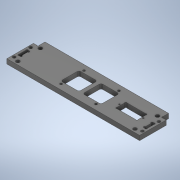
# Autodesk Inventor part: Cockpit_top_frame
Saved by Autodesk Inventor 2020.4 (Build 244396000, 396)
## iProperties
Created: 2022-01-20
Part Number: Cockpit_top_frame
Material: アセタール樹脂、黒
Document SubType Name: Modeling
Designer: Masato Kubotera
Density: 1.425 g/cm^3
Appearance: 滑らか - 黒
Author: Masato Kubotera
Autodesk Inventor part; units mm, degrees
ref_plane "YZ Plane" through (0, 0, 0) normal (1, 0, 0) x (0, 1, 0)
ref_plane "XZ Plane" through (0, 0, 0) normal (0, 1, 0) x (-1, 0, 0)
derived "Cockpit_side_frame.ipt"
sketch "スケッチ1" plane through (0, 0, 0) normal (0, 1, 0) x (-1, 0, 0)
  line L0 (-60, 36.75) -> (60, 36.75) construction
  line L1 (60, 36.75) -> (60, -36.75) construction
  line L2 (60, -36.75) -> (-60, -36.75) construction
  line L3 (-60, -36.75) -> (-60, 36.75) construction
  line L4 (-60, 36.75) -> (60, -36.75) construction
  line L5 (60, 36.75) -> (-60, -36.75) construction
  line L6 (-52.5, 6.75) -> (52.5, 6.75) construction
  line L7 (52.5, 6.75) -> (52.5, 1.75) construction
  line L8 (52.5, 1.75) -> (-52.5, 1.75) construction
  line L9 (-52.5, 1.75) -> (-52.5, 6.75) construction
  line L10 (-52.5, 6.75) -> (52.5, 1.75) construction
  line L11 (52.5, 6.75) -> (-52.5, 1.75) construction
  line L12 (0, 36.75) -> (0, -36.75) construction
  line L13 (-57.5, 34.25) -> (-52.5, 34.25) construction
  line L14 (-52.5, 34.25) -> (-52.5, -34.25) construction
  line L15 (-52.5, -34.25) -> (-57.5, -34.25) construction
  line L16 (-57.5, -34.25) -> (-57.5, 34.25) construction
  line L17 (-57.5, 34.25) -> (-52.5, -34.25) construction
  line L18 (-52.5, 34.25) -> (-57.5, -34.25) construction
  line L19 (-55, 36.75) -> (-60, 31.75)
  line L20 (-60, 0) -> (60, 0) construction
  line L21 (-46.5, 41.75) -> (32.5, 41.75) construction
  line L22 (32.5, 41.75) -> (32.5, 11.75) construction
  line L23 (32.5, 11.75) -> (-46.5, 11.75) construction
  line L24 (-46.5, 11.75) -> (-46.5, 41.75) construction
  line L25 (-46.5, 41.75) -> (32.5, 11.75) construction
  line L26 (32.5, 41.75) -> (-46.5, 11.75) construction
  line L27 (-55, -36.75) -> (-60, -31.75)
  line L28 (-60, 31.75) -> (-60, -31.75)
  line L29 (55, -36.75) -> (60, -31.75)
  line L30 (-52.5, -29.25) -> (52.5, -29.25) construction
  line L31 (52.5, -29.25) -> (52.5, -34.25) construction
  line L32 (52.5, -34.25) -> (-52.5, -34.25) construction
  line L33 (-52.5, -34.25) -> (-52.5, -29.25) construction
  line L34 (-52.5, -29.25) -> (52.5, -34.25) construction
  line L35 (52.5, -29.25) -> (-52.5, -34.25) construction
  line L36 (-25, -29.25) -> (-25, -34.25) construction
  line L37 (-55, -34.25) -> (-55, 34.25) construction
  line L38 (-57.5, 12.5) -> (-52.5, 12.5) construction
  line L39 (-57.55, 12.55) -> (-52.45, 12.55)
  line L40 (-52.45, 12.55) -> (-52.45, -12.55)
  line L41 (-52.45, -12.55) -> (-57.55, -12.55)
  line L42 (-57.55, -12.55) -> (-57.55, 12.55)
  line L43 (-57.55, 12.55) -> (-52.45, -12.55) construction
  line L44 (-52.45, 12.55) -> (-57.55, -12.55) construction
  arc A0 (-52.45, 11.0651) -> (-53.9349, 12.55) centre (-53.1925, 11.8075) ccw
  circle A1 centre (-55, 20) radius 1.6
  circle A2 centre (-55, -20) radius 1.6
  arc A3 (-53.9349, -12.55) -> (-52.45, -11.0651) centre (-53.1925, -11.8075) ccw
  line L45 (-57.5, -12.5) -> (-52.5, -12.5) construction
  arc A4 (-56.0651, 12.55) -> (-57.55, 11.0651) centre (-56.8075, 11.8075) ccw
  arc A5 (-57.55, -11.0651) -> (-56.0651, -12.55) centre (-56.8075, -11.8075) ccw
  line L46 (-52.5, -31.75) -> (52.5, -31.75) construction
  line L47 (-25.05, -34.3) -> (-25.05, -29.2)
  line L48 (-25.05, -29.2) -> (25.05, -29.2)
  circle A6 centre (-32.5, -31.75) radius 1.6
  circle A7 centre (32.5, -31.75) radius 1.6
  line L49 (25, -29.25) -> (25, -34.25) construction
  line L50 (52.5, 36.75) -> (57.5, 36.75) construction
  line L51 (57.5, 36.75) -> (57.5, -34.25) construction
  line L52 (57.5, -34.25) -> (52.5, -34.25) construction
  line L53 (52.5, -34.25) -> (52.5, 36.75) construction
  line L54 (52.5, 36.75) -> (57.5, -34.25) construction
  line L55 (57.5, 36.75) -> (52.5, -34.25) construction
  line L56 (52.5, 1.25) -> (57.5, 1.25) construction
  line L57 (52.5, -11.25) -> (57.5, -11.25) construction
  line L58 (55, -34.25) -> (55, 36.75) construction
  circle A8 centre (55, -18.75) radius 1.6
  line L59 (60, -11.3) -> (52.45, -11.3)
  line L60 (52.45, -11.3) -> (52.45, 13.8)
  arc A9 (52.45, -9.8151) -> (53.9349, -11.3) centre (53.1925, -10.5575) ccw
  line L61 (60, 13.8) -> (52.45, 13.8)
  arc A10 (53.9349, 13.8) -> (52.45, 12.3151) centre (53.1925, 13.0575) ccw
  line L62 (52.5, 13.75) -> (57.5, 13.75) construction
  circle A11 centre (55, 21.25) radius 1.6
  arc A12 (-23.5651, -29.2) -> (-25.05, -30.6849) centre (-24.3075, -29.9425) ccw
  arc A13 (25.05, -30.6849) -> (23.5651, -29.2) centre (24.3075, -29.9425) ccw
  circle A14 centre (-55, 20) radius 3
  circle A15 centre (-32.5, -31.75) radius 3
  circle A16 centre (-55, -20) radius 3
  circle A17 centre (32.5, -31.75) radius 3
  line L63 (25.05, -34.3) -> (25.05, -29.2)
  line L64 (25.05, 6.8) -> (-25.05, 6.8)
  line L65 (-25.05, 6.8) -> (-25.05, 1.7)
  line L66 (-25.05, 1.7) -> (25.05, 1.7)
  line L67 (25.05, 1.7) -> (25.05, 6.8)
  line L68 (25.05, 6.8) -> (-25.05, 1.7) construction
  line L69 (-25.05, 6.8) -> (25.05, 1.7) construction
  line L70 (-25, 6.75) -> (-25, 1.75) construction
  arc A18 (-23.5651, 6.8) -> (-25.05, 5.3151) centre (-24.3075, 6.0575) ccw
  line L71 (52.5, 4.25) -> (-52.5, 4.25) construction
  circle A19 centre (-32.5, 4.25) radius 1.6
  line L72 (25, 6.75) -> (25, 1.75) construction
  arc A20 (25.05, 5.3151) -> (23.5651, 6.8) centre (24.3075, 6.0575) ccw
  circle A21 centre (32.5, 4.25) radius 1.6
  arc A22 (-25.05, 3.1849) -> (-23.5651, 1.7) centre (-24.3075, 2.4425) ccw
  arc A23 (23.5651, 1.7) -> (25.05, 3.1849) centre (24.3075, 2.4425) ccw
  line L73 (60, 31.75) -> (60, 13.8)
  line L74 (60, -11.3) -> (60, -31.75)
  circle A24 centre (-32.5, 4.25) radius 3
  circle A25 centre (55, -18.75) radius 3
  circle A26 centre (55, 21.25) radius 3
  circle A27 centre (32.5, 4.25) radius 3
  line L75 (60, 31.75) -> (60, 39.25)
  line L76 (21, 36.75) -> (-55, 36.75)
  line L77 (60, 39.25) -> (57.5, 41.75)
  line L78 (57.5, 41.75) -> (50, 41.75)
  line L79 (50, 41.75) -> (50, 36.75)
  line L80 (50, 36.75) -> (40.5, 36.75)
  line L81 (40.5, 36.75) -> (40.5, 41.75)
  line L82 (40.5, 41.75) -> (30.5, 41.75)
  line L83 (30.5, 41.75) -> (30.5, 36.75)
  line L84 (30.5, 36.75) -> (21, 36.75)
  line L85 (21, 36.75) -> (21, 36.75)
  circle A28 centre (-45, 4.25) radius 1.75
  line L86 (35.5, 41.75) -> (35.5, 36.75) construction
  line L87 (37.9, -8.6) -> (47.1, -8.6) construction
  line L88 (47.1, -8.6) -> (47.1, -22.4) construction
  line L89 (47.1, -22.4) -> (37.9, -22.4) construction
  line L90 (37.9, -22.4) -> (37.9, -8.6) construction
  line L91 (37.9, -8.6) -> (47.1, -22.4) construction
  line L92 (47.1, -8.6) -> (37.9, -22.4) construction
  line L93 (37.2, -7.95) -> (47.8, -7.95) construction
  line L94 (47.8, -7.95) -> (47.8, -23.05) construction
  line L95 (47.8, -23.05) -> (37.2, -23.05) construction
  line L96 (37.2, -23.05) -> (37.2, -7.95) construction
  line L97 (37.2, -7.95) -> (47.8, -23.05) construction
  line L98 (47.8, -7.95) -> (37.2, -23.05) construction
  line L99 (42.5, -7.95) -> (42.5, -23.05) construction
  line L100 (47.8, -15.5) -> (37.2, -15.5) construction
  line L101 (38.6349, -7.9) -> (46.3651, -7.9)
  line L102 (37.15, -9.3849) -> (37.15, -21.6151)
  line L103 (39.3349, -8.55) -> (45.6651, -8.55)
  line L104 (37.85, -10.0349) -> (37.85, -20.9651)
  arc A29 (38.6349, -7.9) -> (37.15, -9.3849) centre (37.8925, -8.6425) ccw
  arc A30 (39.3349, -8.55) -> (37.85, -10.0349) centre (38.5925, -9.2925) ccw
  arc A31 (47.85, -9.3849) -> (46.3651, -7.9) centre (47.1075, -8.6425) ccw
  arc A32 (47.15, -10.0349) -> (45.6651, -8.55) centre (46.4075, -9.2925) ccw
  line L105 (38.6349, -23.1) -> (46.3651, -23.1)
  line L106 (39.3349, -22.45) -> (45.6651, -22.45)
  arc A33 (37.85, -20.9651) -> (39.3349, -22.45) centre (38.5925, -21.7075) ccw
  arc A34 (37.15, -21.6151) -> (38.6349, -23.1) centre (37.8925, -22.3575) ccw
  arc A35 (46.3651, -23.1) -> (47.85, -21.6151) centre (47.1075, -22.3575) ccw
  arc A36 (45.6651, -22.45) -> (47.15, -20.9651) centre (46.4075, -21.7075) ccw
  line L107 (47.15, -10.0349) -> (47.15, -20.9651)
  line L108 (47.85, -9.3849) -> (47.85, -21.6151)
  line L109 (-45.5, -4.25) -> (10.5, -4.25)
  line L110 (12.5, -6.25) -> (12.5, -22.25)
  line L111 (10.5, -24.25) -> (-45.5, -24.25)
  line L112 (-47.5, -22.25) -> (-47.5, -6.25)
  line L113 (-47.5, -4.25) -> (12.5, -24.25) construction
  line L114 (12.5, -4.25) -> (-47.5, -24.25) construction
  arc A37 (-45.5, -4.25) -> (-47.5, -6.25) centre (-45.5, -6.25) ccw
  arc A38 (-47.5, -22.25) -> (-45.5, -24.25) centre (-45.5, -22.25) ccw
  arc A39 (10.5, -24.25) -> (12.5, -22.25) centre (10.5, -22.25) ccw
  arc A40 (12.5, -6.25) -> (10.5, -4.25) centre (10.5, -6.25) ccw
  line L115 (26.5, 36.75) -> (26.5, 32.75) construction
  line L116 (24.5, 32.75) -> (28.5, 32.75) construction
  line L117 (28.5, 32.75) -> (28.5, 36.75) construction
  line L118 (24.5, 32.75) -> (24.5, 36.75) construction
  line L119 (42.5, 32.75) -> (42.5, 36.75) construction
  line L120 (44.5, 36.75) -> (44.5, 32.75) construction
  line L121 (46.5, 32.75) -> (42.5, 32.75) construction
  line L122 (46.5, 32.75) -> (46.5, 36.75) construction
  arc A41 (48.5151, 36.75) -> (50, 38.2349) centre (49.2575, 37.4925) ccw
  arc A42 (29.0151, 36.75) -> (30.5, 38.2349) centre (29.7575, 37.4925) ccw
  arc A43 (40.5, 38.2349) -> (41.9849, 36.75) centre (41.2425, 37.4925) ccw
  line L123 (30.5, 36.75) -> (40.5, 36.75)
  line L124 (60, -36.75) -> (60, -79.25)
  line L125 (60, -79.25) -> (14, -79.25)
  line L126 (9, -74.25) -> (9, -36.75)
  arc A44 (-25.05, -32.8151) -> (-23.5651, -34.3) centre (-24.3075, -33.5575) ccw
  arc A45 (23.5651, -34.3) -> (25.05, -32.8151) centre (24.3075, -33.5575) ccw
  line L127 (60, -36.75) -> (60, -31.75)
  line L128 (-25.05, -34.3) -> (25.05, -34.3)
  line L129 (-55, -36.75) -> (9, -36.75)
  line L130 (16.5, -48.75) -> (50.5, -48.75) construction
  line L131 (50.5, -48.75) -> (50.5, -71.75) construction
  line L132 (50.5, -71.75) -> (16.5, -71.75) construction
  line L133 (16.5, -71.75) -> (16.5, -48.75) construction
  line L134 (16.5, -48.75) -> (50.5, -71.75) construction
  line L135 (50.5, -48.75) -> (16.5, -71.75) construction
  line L136 (14, -45.5) -> (16.5, -45.5) construction
  line L137 (16.5, -45.5) -> (16.5, -60.5) construction
  line L138 (16.5, -60.5) -> (14, -60.5) construction
  line L139 (14, -60.5) -> (14, -45.5) construction
  line L140 (14, -45.5) -> (16.5, -60.5) construction
  line L141 (16.5, -45.5) -> (14, -60.5) construction
  line L142 (13.95, -45.45) -> (16.55, -45.45)
  line L143 (16.55, -45.45) -> (16.55, -60.55)
  line L144 (16.55, -60.55) -> (13.95, -60.55)
  line L145 (13.95, -60.55) -> (13.95, -45.45)
  line L146 (13.95, -45.45) -> (16.55, -60.55) construction
  line L147 (16.55, -45.45) -> (13.95, -60.55) construction
  line L148 (15.25, -45.5) -> (15.25, -60.5) construction
  line L149 (14, -53) -> (16.5, -53) construction
  arc A46 (15.4349, -45.45) -> (13.95, -46.9349) centre (14.6925, -46.1925) ccw
  arc A47 (16.55, -47.55) -> (16.55, -45.45) centre (16.55, -46.5) ccw
  arc A48 (13.95, -59.0651) -> (15.4349, -60.55) centre (14.6925, -59.8075) ccw
  arc A49 (16.55, -60.55) -> (16.55, -58.45) centre (16.55, -59.5) ccw
  line L150 (11.5, -34.25) -> (16.5, -34.25) construction
  line L151 (16.5, -34.25) -> (16.5, -71.75) construction
  line L152 (16.5, -71.75) -> (11.5, -71.75) construction
  line L153 (11.5, -71.75) -> (11.5, -34.25) construction
  line L154 (11.5, -34.25) -> (16.5, -71.75) construction
  line L155 (16.5, -34.25) -> (11.5, -71.75) construction
  circle A50 centre (14, -39.5) radius 1.6
  line L156 (14, -34.25) -> (14, -71.75) construction
  circle A51 centre (14, -66.5) radius 1.6
  line L157 (14, -79.25) -> (9, -74.25)
  circle A52 centre (14, -39.5) radius 3
  circle A53 centre (14, -66.5) radius 3
  line L158 (11.5, -71.75) -> (50, -71.75) construction
  line L159 (50, -71.75) -> (50, -76.75) construction
  line L160 (50, -76.75) -> (11.5, -76.75) construction
  line L161 (11.5, -76.75) -> (11.5, -71.75) construction
  line L162 (11.5, -71.75) -> (50, -76.75) construction
  line L163 (50, -71.75) -> (11.5, -76.75) construction
  line L164 (30.75, -76.75) -> (30.75, -71.75) construction
  line L165 (11.5, -74.25) -> (50, -74.25) construction
  line L166 (25.75, -71.75) -> (35.75, -71.75) construction
  line L167 (35.75, -71.75) -> (35.75, -74.25) construction
  line L168 (35.75, -74.25) -> (25.75, -74.25) construction
  line L169 (25.75, -74.25) -> (25.75, -71.75) construction
  line L170 (25.75, -71.75) -> (35.75, -74.25) construction
  line L171 (35.75, -71.75) -> (25.75, -74.25) construction
  line L172 (25.7, -71.7) -> (35.8, -71.7)
  line L173 (35.8, -71.7) -> (35.8, -74.3)
  line L174 (35.8, -74.3) -> (25.7, -74.3)
  line L175 (25.7, -74.3) -> (25.7, -71.7)
  line L176 (25.7, -71.7) -> (35.8, -74.3) construction
  line L177 (35.8, -71.7) -> (25.7, -74.3) construction
  arc A54 (25.7, -72.8151) -> (27.1849, -74.3) centre (26.4425, -73.5575) ccw
  arc A55 (27.8, -71.7) -> (25.7, -71.7) centre (26.75, -71.7) ccw
  arc A56 (34.3151, -74.3) -> (35.8, -72.8151) centre (35.0575, -73.5575) ccw
  arc A57 (35.8, -71.7) -> (33.7, -71.7) centre (34.75, -71.7) ccw
  circle A58 centre (42.75, -74.25) radius 1.6
  circle A59 centre (42.75, -74.25) radius 3
  point P0 (0, 0)
  point P1 (0, 4.25)
  point P2 (-55, 0)
  point P3 (-55, 0)
  point P4 (-7, 26.75)
  point P5 (0, -31.75)
  point P6 (-25.05, -34.25)
  point P7 (25.05, -34.25)
  point P8 (0, 4.25)
  point P9 (42.5, -15.5)
  point P10 (37.15, -7.9)
  point P11 (37.85, -8.55)
  point P12 (-17.5, -14.25)
  point P13 (9, -79.25)
  point P14 (33.5, -60.25)
  point P15 (15.25, -53)
  point P16 (30.75, -74.25)
  point P17 (30.75, -73)
  dimension "d1" = 36.75
  dimension "d4" = 29
  dimension "d5" = 18
  dimension "d6" = 10
  dimension "d28" = 36.5
  measures "d1" vertical distance of point (0, 0) L0.end
  measures "d4" distance of L79.end L76.start
  measures "d5" distance of L120.start L115.start
  measures "d6" distance of L81.end L82.end
  measures "d28" horizontal distance of L76.start L77.end
ref_plane "作業平面1" through (0, 0, 36.75) normal (0, 0, 1) x (1, 0, 0)
sketch "スケッチ2" plane through (0, 0, 36.75) normal (0, 0, 1) x (1, 0, 0)
  line L0 (-21, -144.5) -> (-57.5, -144.5) construction
  line L1 (-57.5, -144.5) -> (-57.5, 0) construction
  line L2 (-57.5, 0) -> (-21, 0) construction
  line L3 (-21, 0) -> (-21, -144.5)
  line L4 (-40.5, -2.5) -> (-30.5, -2.5) construction
  line L5 (-30.5, -2.5) -> (-30.5, -5) construction
  line L6 (-30.5, -5) -> (-40.5, -5) construction
  line L7 (-40.5, -5) -> (-40.5, -2.5) construction
  line L8 (-40.5, -2.5) -> (-30.5, -5) construction
  line L9 (-30.5, -2.5) -> (-40.5, -5) construction
  line L10 (-35.5, -2.5) -> (-35.5, -5) construction
  line L11 (-40.55, -2.45) -> (-30.45, -2.45)
  line L12 (-30.45, -2.45) -> (-30.45, -5.05)
  line L13 (-30.45, -5.05) -> (-40.55, -5.05)
  line L14 (-40.55, -5.05) -> (-40.55, -2.45)
  line L15 (-40.55, -2.45) -> (-30.45, -5.05) construction
  line L16 (-30.45, -2.45) -> (-40.55, -5.05) construction
  line L17 (-40.5, -3.75) -> (-30.5, -3.75) construction
  circle A0 centre (-44.5, -2.5) radius 1.6
  circle A1 centre (-26.5, -2.5) radius 1.6
  arc A2 (-39.0651, -2.45) -> (-40.55, -3.9349) centre (-39.8075, -3.1925) ccw
  arc A3 (-40.55, -5.05) -> (-38.45, -5.05) centre (-39.5, -5.05) ccw
  arc A4 (-30.45, -3.9349) -> (-31.9349, -2.45) centre (-31.1925, -3.1925) ccw
  arc A5 (-32.55, -5.05) -> (-30.45, -5.05) centre (-31.5, -5.05) ccw
  line L18 (-49.95, 0) -> (-49.95, -3.5151)
  line L19 (-51.4349, -5) -> (-57.5, -5)
  arc A6 (-51.4349, -5) -> (-49.95, -3.5151) centre (-50.6925, -4.2575) ccw
  line L20 (-50, 0) -> (-21, 0)
  line L21 (-57.5, -72.25) -> (-21, -72.25) construction
  line L22 (-40.55, -142.05) -> (-30.45, -142.05)
  line L23 (-30.45, -142.05) -> (-30.45, -139.45)
  line L24 (-30.45, -139.45) -> (-40.55, -139.45)
  line L25 (-40.55, -139.45) -> (-40.55, -142.05)
  circle A7 centre (-44.5, -142) radius 1.6
  circle A8 centre (-26.5, -142) radius 1.6
  arc A9 (-40.55, -140.5651) -> (-39.0651, -142.05) centre (-39.8075, -141.3075) ccw
  arc A10 (-38.45, -139.45) -> (-40.55, -139.45) centre (-39.5, -139.45) ccw
  arc A11 (-31.9349, -142.05) -> (-30.45, -140.5651) centre (-31.1925, -141.3075) ccw
  arc A12 (-30.45, -139.45) -> (-32.55, -139.45) centre (-31.5, -139.45) ccw
  line L26 (-49.95, -144.5) -> (-49.95, -140.9849)
  line L27 (-51.4349, -139.5) -> (-57.5, -139.5)
  arc A13 (-49.95, -140.9849) -> (-51.4349, -139.5) centre (-50.6925, -140.2425) ccw
  line L28 (-50, -144.5) -> (-21, -144.5)
  line L29 (-57.5, -139.5) -> (-57.5, -5)
  line L30 (-29.9, -69.6) -> (-48.6, -69.6) construction
  line L31 (-48.6, -69.6) -> (-48.6, -50.9) construction
  line L32 (-48.6, -50.9) -> (-29.9, -50.9) construction
  line L33 (-29.9, -50.9) -> (-29.9, -69.6) construction
  line L34 (-29.9, -69.6) -> (-48.6, -50.9) construction
  line L35 (-48.6, -69.6) -> (-29.9, -50.9) construction
  line L36 (-39.25, -60.25) -> (-39.25, -84.25) construction
  line L37 (-31.3142, -50.3142) -> (-47.1858, -50.3142)
  line L38 (-49.1858, -52.3142) -> (-49.1858, -68.1858)
  line L39 (-47.1858, -70.1858) -> (-31.3142, -70.1858)
  line L40 (-29.3142, -68.1858) -> (-29.3142, -52.3142)
  line L41 (-29.3142, -50.3142) -> (-49.1858, -70.1858) construction
  line L42 (-49.1858, -50.3142) -> (-29.3142, -70.1858) construction
  arc A14 (-29.3142, -52.3142) -> (-31.3142, -50.3142) centre (-31.3142, -52.3142) ccw
  arc A15 (-47.1858, -50.3142) -> (-49.1858, -52.3142) centre (-47.1858, -52.3142) ccw
  arc A16 (-49.1858, -68.1858) -> (-47.1858, -70.1858) centre (-47.1858, -68.1858) ccw
  arc A17 (-31.3142, -70.1858) -> (-29.3142, -68.1858) centre (-31.3142, -68.1858) ccw
  line L43 (-31.3142, -94.1858) -> (-47.1858, -94.1858)
  line L44 (-49.1858, -92.1858) -> (-49.1858, -76.3142)
  line L45 (-47.1858, -74.3142) -> (-31.3142, -74.3142)
  line L46 (-29.3142, -76.3142) -> (-29.3142, -92.1858)
  arc A18 (-31.3142, -94.1858) -> (-29.3142, -92.1858) centre (-31.3142, -92.1858) ccw
  arc A19 (-49.1858, -92.1858) -> (-47.1858, -94.1858) centre (-47.1858, -92.1858) ccw
  arc A20 (-47.1858, -74.3142) -> (-49.1858, -76.3142) centre (-47.1858, -76.3142) ccw
  arc A21 (-29.3142, -76.3142) -> (-31.3142, -74.3142) centre (-31.3142, -76.3142) ccw
  line L47 (-26.75, -53.25) -> (-51.75, -53.25) construction
  line L48 (-51.75, -53.25) -> (-51.75, -91.25) construction
  line L49 (-51.75, -91.25) -> (-26.75, -91.25) construction
  line L50 (-26.75, -91.25) -> (-26.75, -53.25) construction
  line L51 (-26.75, -53.25) -> (-51.75, -91.25) construction
  line L52 (-51.75, -53.25) -> (-26.75, -91.25) construction
  circle A22 centre (-26.75, -53.25) radius 1.25
  circle A23 centre (-51.75, -53.25) radius 1.25
  circle A24 centre (-26.75, -91.25) radius 1.25
  circle A25 centre (-51.75, -91.25) radius 1.25
  line L53 (-34, -16) -> (-44.5, -16) construction
  line L54 (-44.5, -16) -> (-44.5, -38.5) construction
  line L55 (-44.5, -38.5) -> (-34, -38.5) construction
  line L56 (-34, -38.5) -> (-34, -16) construction
  line L57 (-34, -16) -> (-44.5, -38.5) construction
  line L58 (-44.5, -16) -> (-34, -38.5) construction
  line L59 (-39.25, -14.25) -> (-39.25, -40.25) construction
  line L60 (-34, -27.25) -> (-44.5, -27.25) construction
  circle A26 centre (-39.25, -14.25) radius 0.75
  circle A27 centre (-39.25, -40.25) radius 0.75
  line L61 (-33.75, -15.75) -> (-44.75, -15.75)
  line L62 (-44.75, -15.75) -> (-44.75, -38.75)
  line L63 (-44.75, -38.75) -> (-33.75, -38.75)
  line L64 (-33.75, -38.75) -> (-33.75, -15.75)
  line L65 (-33.75, -15.75) -> (-44.75, -38.75) construction
  line L66 (-44.75, -15.75) -> (-33.75, -38.75) construction
  arc A28 (-33.75, -17.2349) -> (-35.2349, -15.75) centre (-34.4925, -16.4925) ccw
  arc A29 (-35.2349, -38.75) -> (-33.75, -37.2651) centre (-34.4925, -38.0075) ccw
  arc A30 (-43.2651, -15.75) -> (-44.75, -17.2349) centre (-44.0075, -16.4925) ccw
  arc A31 (-44.75, -37.2651) -> (-43.2651, -38.75) centre (-44.0075, -38.0075) ccw
  line L67 (-24.5, -8.5) -> (-49, -8.5) construction
  line L68 (-49, -8.5) -> (-49, -136) construction
  line L69 (-49, -136) -> (-24.5, -136) construction
  line L70 (-24.5, -136) -> (-24.5, -8.5) construction
  circle A32 centre (-24.5, -8.5) radius 2
  circle A33 centre (-49, -8.5) radius 2
  circle A34 centre (-24.5, -136) radius 2
  circle A35 centre (-49, -136) radius 2
  point P0 (0, 0)
  point P1 (-35.5, 0)
  point P2 (-35.5, 0)
  point P3 (-35.5, 0)
  point P4 (-60, 0)
  point P5 (-35.5, -3.75)
  point P6 (-49.95, -5)
  point P7 (-30.45, -140.5651)
  point P8 (-31.9349, -142.05)
  point P9 (-32.55, -5.05)
  point P10 (-31.9349, -2.45)
  point P11 (-30.45, -3.9349)
  point P12 (-39.25, -72.25)
  point P13 (-39.25, -27.25)
  point P14 (-39.25, -27.25)
  point P15 (-43.2651, -38.75)
  point P16 (-44.75, -17.2349)
  dimension "d8" = 36.5
  dimension "d10" = 144.5
  dimension "d11" = 10
  dimension "d12" = 2.5
  dimension "d14" = 3.2
  dimension "d16" = 2.5
  dimension "d17" = 18
  dimension "d18" = 1.05
  dimension "d19" = 1.05
  dimension "d20" = 0.05
  dimension "d21" = 0.05
  dimension "d23" = 0.05
  dimension "d24" = 1.05
  dimension "d25" = 5
  dimension "d29" = 18.7
  dimension "d30" = 18.7
  dimension "d31" = 24
  dimension "d32" = 2
  dimension "d33" = 18.25
  dimension "d34" = 25
  dimension "d35" = 38
  dimension "d36" = 2.5
  dimension "d37" = 2.5
  dimension "d38" = 10.5
  dimension "d39" = 22.5
  dimension "d40" = 26
  dimension "d41" = 1.5
  dimension "d43" = 45
  dimension "d44" = 1.05
  dimension "d45" = 23
  dimension "d46" = 11
  dimension "d47" = 3.5
  dimension "d48" = 3.5
  dimension "d49" = 4
  dimension "d50" = 4
  dimension "d51" = 8.5
  constraints: 142 end point, 55 symmetric about line, 49 point on circle, 36 centre point, 26 midpoint, 23 point on line, 18 parallel, 10 horizontal, 10 perpendicular, 8 tangent, 6 coincident, 3 collinear, 3 equal radius, 3 vertical, 22 other
  measures "d8" distance of L1.end L2.end
  measures "d10" distance of L0.end L1.end
  measures "d11" distance of L5.end L6.end
  measures "d12" distance of L4.end L5.end
  measures "d14" diameter of A0
  measures "d16" vertical distance of A0.centre point (-35.5, 0)
  measures "d17" distance of A1.centre A0.centre
  measures "d18" radius of A2
  measures "d19" radius of A3
  measures "d20" horizontal distance of L11.start L4.start
  measures "d21" horizontal distance of L11.start L4.start
  measures "d23" distance of L18.start point (-50, 0)
  measures "d24" radius of A6
  measures "d25" distance from line of L19 L18.start
  measures "d29" distance of L32.end L31.end
  measures "d30" distance of L30.end L31.end
  measures "d31" distance of L36.start L36.end
  measures "d32" radius of A14
  measures "d33" distance of L21.end point (-39.25, -72.25)
  measures "d34" distance of L49.end L48.end
  measures "d35" distance of L48.end L47.end
  measures "d36" diameter of A22
  measures "d37" diameter of A23
  measures "d38" distance of L55.end L54.end
  measures "d39" distance of L54.end L53.end
  measures "d40" distance of L59.start L59.end
  measures "d41" diameter of A26
  measures "d43" vertical distance of L21.end L60.start
  measures "d44" radius of A28
  measures "d45" distance of L63.end L61.start
  measures "d46" distance of L61.start L61.end
  measures "d47" horizontal distance of L2.end L67.start
  measures "d48" vertical distance of L19.end L67.end
  measures "d49" diameter of A32
  measures "d50" diameter of A33
  measures "d51" horizontal distance of L19.end L67.end
extrude "押し出し1" add sketch "スケッチ2" along normal blind 5
equation "\"d8\" = d28"
equation "\"d11\" = d6"
equation "\"d16\" = 0.5 * d22"
equation "\"d17\" = d5"
equation "\"d19\" = d18"
equation "\"d21\" = d20"
equation "\"d23\" = d20"
equation "\"d24\" = d18"
equation "\"d29\" = d30"
equation "\"d33\" = 0.5 * d8"
equation "\"d37\" = d36"
equation "\"d48\" = d47"
equation "\"d50\" = d49"
equation "\"d7\" = d1"
equation "\"d22\" = 5"
